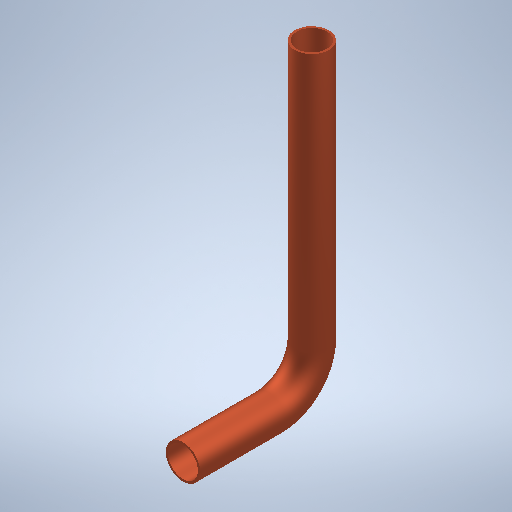
# Autodesk Inventor part: Auspuffkrümmer
Saved by Autodesk Inventor 2025 (Build 290162010, 162A)
## iProperties
Created: 2024-04-30
Part Number: Auspuffkrümmer
Material: Copper, Cast
Document SubType Name: Modeling
Designer: ffogue
Density: 8.94 g/cm^3
Appearance: Copper - Satin
Author: ffogue
Autodesk Inventor part; units mm, degrees
ref_plane "XZ Plane" through (0, 0, 0) normal (0, 1, 0) x (-1, 0, 0)
ref_plane "XY Plane" through (0, 0, 0) normal (0, 0, 1) x (1, 0, 0)
sketch "Skizze1" plane through (0, 0, 0) normal (0, 1, 0) x (-1, 0, 0)
  circle A0 centre (0, 0) radius 4
  circle A1 centre (0, 0) radius 3.5
  dimension "d0" = 8
  dimension "d1" = 7
  constraints: 2 centre point, 2 coincident
  measures "d0" diameter of A0
  measures "d1" diameter of A1
ref_plane "Arbeitsebene1" through (0, 0, 0) normal (1, 0, 0) x (0, 1, 0)
sketch "Skizze2" plane through (0, 0, 0) normal (1, 0, 0) x (0, 1, 0)
  line L0 (0, 0) -> (20, 0)
  line L1 (30, 10) -> (30, 70)
  arc A0 (20, 0) -> (30, 10) centre (20, 10) ccw
  point P0 (30, 0)
  dimension "d3" = 70
  dimension "d4" = 10
  dimension "d5" = 30
  constraints: 4 end point, 2 point on circle, 2 point on line, 2 tangent, 1 centre point, 1 horizontal, 1 perpendicular
  measures "d3" distance of point (30, 0) L1.end
  measures "d4" radius of A0
  measures "d5" distance from line of L0.start L1
sweep "Sweeping1" add profiles "Skizze1" path "Skizze2"
